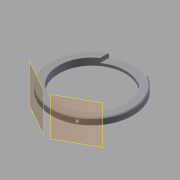
# Autodesk Inventor part: KE-SP-02-P1
Saved by Autodesk Inventor 2018 (Build 220112000, 112)
## iProperties
Created: 2015-08-04
Part Number: KE-SP-02-P1
Material: 一般
Document SubType Name: Modeling
Designer: ERIC
Density: 1 g/cm^3
Appearance: 預設
Author: ERIC
Autodesk Inventor part; units mm, degrees
ref_plane "YZ Plane" through (0, 0, 0) normal (1, 0, 0) x (0, 1, 0)
ref_plane "XZ Plane" through (0, 0, 0) normal (0, 1, 0) x (-1, 0, 0)
sketch "草圖1" plane through (0, 0, 0) normal (0, 0, 1) x (1, 0, 0)
  circle A0 centre (0, 0) radius 19.05
  circle A1 centre (0, 0) radius 23.35
  dimension "d0" = 38.1
  dimension "d3" = 46.7
  constraints: 2 centre point, 2 coincident
  measures "d0" diameter of A0
  measures "d3" diameter of A1
extrude "擠出1" add sketch "草圖1" along normal blind 4
sketch "草圖2" plane through (0, 0, 4) normal (0, 0, 1) x (1, 0, 0)
  circle A0 centre (0, 0) radius 23.35 projected
  line L0 (11, 28.8223) -> (11, 20.5967)
  line L1 (-11, 28.8223) -> (-11, 20.5967)
  line L2 (-11, 28.8223) -> (11, 28.8223)
  line L3 (11, 28.8223) -> (11, 13.5331)
  line L4 (11, 13.5331) -> (-11, 13.5331)
  line L5 (-11, 13.5331) -> (-11, 28.8223)
  circle A1 centre (0, 0) radius 19.05 construction
  circle A2 centre (0, 0) radius 23.35 construction
  line L6 (0, 0) -> (0, 44.5236) construction
  dimension "d6" = 22
  dimension "d27" = 11
  dimension "d28" = 11
  constraints: 14 end point, 3 parallel, 2 point on circle, 2 vertical, 1 horizontal, 1 perpendicular, 1 other
  measures "d6" distance between parallel lines of L0 L1
  measures "d27" distance between parallel lines of L0 L6
  measures "d28" horizontal distance of A0.centre L0.end
extrude "擠出2" cut sketch "草圖2" against normal blind 2.5 contours L3 L4 L5 A0 | A0 L1 L2 L0 picked at (0, 16.8054)
ref_plane "工作平面1" through (0, 0, 2) normal (0, 0, 1) x (1, 0, 0)
sketch "草圖3" plane through (0, 0, 2) normal (0, 0, 1) x (1, 0, 0)
  line L0 (0, 0) -> (0, -42.4806)
  line L1 (0, 0) -> (-11.5, -20.325)
  line L2 (0, 0) -> (11.5, -20.325)
  line L3 (-11.5, -20.325) -> (11.5, -20.325)
  line L4 (11, 20.5967) -> (11, 15.5532) construction
  arc A0 (-11, 15.5532) -> (11, 15.5532) centre (0, 0) ccw construction
  line L5 (-11, 15.5532) -> (-11, 20.5967) construction
  arc A1 (-11, 20.5967) -> (11, 20.5967) centre (0, 0) ccw construction
  dimension "d9" = 23
  dimension "d29" = 59.003
  dimension "d31" = 20.325
  dimension "d38" = 29.501
  constraints: 8 end point, 1 perpendicular, 1 vertical, 1 other
  measures "d9" distance of L1.end L2.end
  measures "d29" angle of L1 L2
  measures "d31" distance from line of A1.centre L3
  measures "d38" angle of L0 L2
chamfer "倒角1" distance 0.5 angle 45 3 edges at (-12.0078, -20.0259, 4) (20.0259, 12.0078, 4) (-23.35, 0, 0)
ref_plane "工作平面5" through (-11.5, -20.325, 2) normal (-0.4924452, -0.8703434, 0) x (0.8703434, -0.4924452, 0)
ref_plane "工作平面6" through (11.5, -20.325, 2) normal (0.4924452, -0.8703434, 0) x (0.8703434, 0.4924452, 0)
sketch "草圖6" plane through (11.5, -20.325, 2) normal (0.4924452, -0.8703434, 0) x (0.8703434, 0.4924452, 0)
  circle A0 centre (0, 0) radius 1
  point P0 (0, -2)
  dimension "d32" = 2
  constraints: 1 centre point
  measures "d32" diameter of A0
extrude "擠出3" cut sketch "草圖6" against normal blind 2.5
sketch "草圖7" plane through (-11.5, -20.325, 2) normal (-0.4924452, -0.8703434, 0) x (0.8703434, -0.4924452, 0)
  circle A0 centre (0, 0) radius 1
  point P0 (0, -2)
  dimension "d35" = 2
  constraints: 1 centre point
  measures "d35" diameter of A0
extrude "擠出4" cut sketch "草圖7" against normal blind 2.5
equation "\"d27\" = 0.5 * d6"
